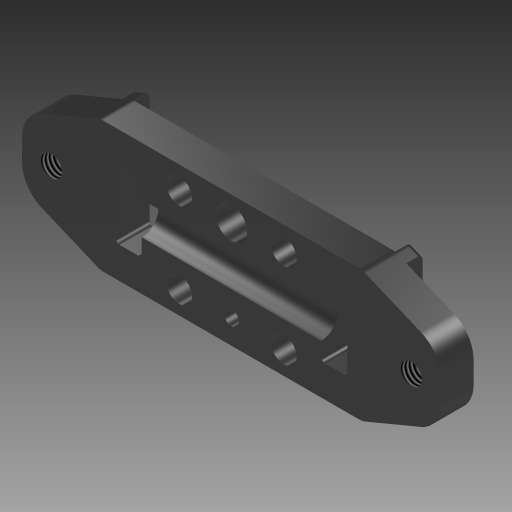
# Autodesk Inventor part: TTB Sliding Bearing Block Plate (SLIDE-001)
Saved by Autodesk Inventor 2023 (Build 270158000, 158)
## iProperties
Created: 2022-11-17
Part Number: TTB Sliding Bearing Block Plate (SLIDE-001)
Material: Aluminum 6061
Document SubType Name: Modeling
Designer: Max Boord
Mass: 26.5057 g
Surface Area: 60.4587 cm^2
Volume: 9.81693 cm^3
Density: 2.7 g/cm^3
Appearance: Glossy - Black
Author: Max Boord
Autodesk Inventor part; units mm, degrees
ref_plane "YZ Plane" through (0, 0, 0) normal (1, 0, 0) x (0, 1, 0)
ref_plane "XZ Plane" through (0, 0, 0) normal (0, 1, 0) x (-1, 0, 0)
ref_plane "XY Plane" through (0, 0, 0) normal (0, 0, 1) x (1, 0, 0)
sketch "Sketch1" plane through (0, 0, 0) normal (0, 0, 1) x (1, 0, 0)
  arc A0 (24.765, -12.7) -> (25.9862, -12.4558) centre (24.765, -9.525) ccw
  line L0 (25.9862, -12.4558) -> (36.7323, -7.9782)
  arc A1 (36.7323, -7.9782) -> (40.64, -2.1167) centre (34.29, -2.1167) ccw
  line L1 (40.64, -2.1167) -> (40.64, 2.1167)
  arc A2 (40.64, 2.1167) -> (36.7323, 7.9782) centre (34.29, 2.1167) ccw
  line L2 (36.7323, 7.9782) -> (25.9862, 12.4558)
  arc A3 (25.9862, 12.4558) -> (24.765, 12.7) centre (24.765, 9.525) ccw
  line L3 (24.765, 12.7) -> (-24.765, 12.7)
  arc A4 (-24.765, 12.7) -> (-25.9862, 12.4558) centre (-24.765, 9.525) ccw
  line L4 (-25.9862, 12.4558) -> (-36.7323, 7.9782)
  arc A5 (-36.7323, 7.9782) -> (-40.64, 2.1167) centre (-34.29, 2.1167) ccw
  line L5 (-40.64, 2.1167) -> (-40.64, -2.1167)
  arc A6 (-40.64, -2.1167) -> (-36.7323, -7.9782) centre (-34.29, -2.1167) ccw
  line L6 (-36.7323, -7.9782) -> (-25.9862, -12.4558)
  arc A7 (-25.9862, -12.4558) -> (-24.765, -12.7) centre (-24.765, -9.525) ccw
  line L7 (-24.765, -12.7) -> (24.765, -12.7)
  circle A8 centre (0, -7.9502) radius 1.4605
  circle A9 centre (-34.925, 0) radius 2.0193
  circle A10 centre (34.925, 0) radius 2.0193
  circle A11 centre (-10.16, 8.255) radius 2.4892
  circle A12 centre (-10.16, -8.255) radius 2.4892
  circle A13 centre (10.16, 8.255) radius 2.4892
  circle A14 centre (10.16, -8.255) radius 2.4892
  line L8 (17.399, -3.1979) -> (-17.399, -3.1979)
  line L9 (-17.399, -3.1979) -> (-17.399, -5.7785)
  arc A15 (-18.2245, -6.604) -> (-17.399, -5.7785) centre (-18.2245, -5.7785) ccw
  line L10 (-18.2245, -6.604) -> (-21.6535, -6.604)
  arc A16 (-22.479, -5.7785) -> (-21.6535, -6.604) centre (-21.6535, -5.7785) ccw
  line L11 (-22.479, -5.7785) -> (-22.479, 5.7785)
  arc A17 (-21.6535, 6.604) -> (-22.479, 5.7785) centre (-21.6535, 5.7785) ccw
  line L12 (-21.6535, 6.604) -> (-18.2245, 6.604)
  arc A18 (-17.399, 5.7785) -> (-18.2245, 6.604) centre (-18.2245, 5.7785) ccw
  line L13 (-17.399, 5.7785) -> (-17.399, 3.1979)
  line L14 (-17.399, 3.1979) -> (17.399, 3.1979)
  line L15 (17.399, 3.1979) -> (17.399, 5.7785)
  arc A19 (18.2245, 6.604) -> (17.399, 5.7785) centre (18.2245, 5.7785) ccw
  line L16 (18.2245, 6.604) -> (21.6535, 6.604)
  arc A20 (22.479, 5.7785) -> (21.6535, 6.604) centre (21.6535, 5.7785) ccw
  line L17 (22.479, 5.7785) -> (22.479, -5.7785)
  arc A21 (21.6535, -6.604) -> (22.479, -5.7785) centre (21.6535, -5.7785) ccw
  line L18 (21.6535, -6.604) -> (18.2245, -6.604)
  arc A22 (17.399, -5.7785) -> (18.2245, -6.604) centre (18.2245, -5.7785) ccw
  line L19 (17.399, -5.7785) -> (17.399, -3.1979)
  circle A23 centre (0, 7.9502) radius 3.048
  line L20 (-40.64, 0) -> (40.64, 0) construction
  line L21 (0, 7.9502) -> (0, -7.9502) construction
  line L22 (-10.16, 8.255) -> (10.16, -8.255) construction
  line L23 (-10.16, -8.255) -> (10.16, 8.255) construction
  line L24 (-34.925, 0) -> (0, 0) construction
  line L25 (0, 0) -> (34.925, 0) construction
  line L26 (-25.4, 12.6359) -> (-25.4, -12.6359)
  line L27 (-27.6098, -11.7792) -> (-27.6098, 11.7792)
  line L28 (27.6098, 11.7792) -> (27.6098, -11.7792)
  line L29 (25.4, -12.6359) -> (25.4, 12.6359)
  line L30 (-17.399, 3.1979) -> (-17.399, -3.1979)
  line L31 (17.399, 3.1979) -> (17.399, -3.1979)
  line L32 (0, 7.9502) -> (0, -7.9502) construction
  line L33 (-1.4605, 7.9502) -> (-1.4605, -7.9502)
  line L34 (1.4605, -7.9502) -> (1.4605, 7.9502)
  arc A24 (1.4605, 7.9502) -> (-1.4605, 7.9502) centre (0, 7.9502) ccw
  arc A25 (-1.4605, -7.9502) -> (1.4605, -7.9502) centre (0, -7.9502) ccw
  point P0 (0, 12.7)
  point P1 (0, -12.7)
  point P2 (0, -3.1979)
  point P3 (0, 3.1979)
  point P4 (-22.479, 0)
  point P5 (22.479, 0)
  dimension "d0" = 4.9784
  dimension "d1" = 69.85
  dimension "d2" = 25.4
  dimension "d3" = 81.28
  dimension "d4" = 16.51
  dimension "d5" = 20.32
  dimension "d6" = 15.9004
  dimension "d7" = 13.208
  dimension "d8" = 5.08
  dimension "d9" = 1.651
  dimension "d11" = 6.3958
  dimension "d12" = 44.958
  dimension "d13" = 4.0386
  dimension "d14" = 6.35
  dimension "d15" = 4.2333
  dimension "d16" = 49.53
  dimension "d17" = 3.175
  dimension "d18" = 2.921
  dimension "d19" = 6.096
  dimension "d21" = 50.8
  dimension "d22" = 2.2098
  constraints: 72 end point, 49 centre point, 40 point on circle, 36 tangent, 18 equal radius, 13 midpoint, 12 equal length, 7 horizontal, 6 point on line, 4 horizontal alignment, 4 parallel, 4 perpendicular, 4 vertical, 3 vertical alignment, 1 coincident, 1 collinear, 3 other
  measures "d0" diameter of A11
  measures "d1" distance of L25.end L24.start
  measures "d2" distance between parallel lines of L7 L3
  measures "d3" distance between parallel lines of L1 L5
  measures "d4" distance of L23.start L22.start
  measures "d5" distance of L23.end L22.start
  measures "d6" distance of L21.end L21.start
  measures "d7" distance between parallel lines of L10 L12
  measures "d8" distance between parallel lines of L13 L11
  measures "d9" diameter of A17
  measures "d11" distance between parallel lines of L14 L8
  measures "d12" distance between parallel lines of L11 L17
  measures "d13" diameter of A9
  measures "d14" radius of A2
  measures "d15" distance of L5.start L5.end
  measures "d16" distance of L3.start L3.end
  measures "d17" radius of A4
  measures "d18" diameter of A8
  measures "d19" diameter of A23
  measures "d21" distance between parallel lines of L29 L26
  measures "d22" distance between parallel lines of L29 L28
extrude "Extrusion1" add sketch "Sketch1" along normal blind 6.35 contours L7 A7 L26 A4 L3 A3 L29 A0 | L29 A3 L2 L28 L0 A0 | A7 L6 L27 L4 A4 L26 | L28 L2 A2 L1 A1 L0 | L6 A6 L5 A5 L4 L27 | A8 L33 L8 L34 | L34 L14 L31 L8 | L8 L33 L14 L34 | L8 L30 L14 L33 | L14 L33 A23 L34 | L34 A24 L33 A23 | A23 L33 A24 L34
extrude "Extrusion2" add sketch "Sketch1" against normal blind 3.175 contours L29 A3 L2 L28 L0 A0 | A7 L6 L27 L4 A4 L26
extrude "Extrusion3" cut sketch "Sketch1" against normal blind 3.1979 from surface at 6.35 contours L34 L14 L31 L8 | L8 L33 L14 L34 | L8 L30 L14 L33
full round fillet "Full Round Fillet1" first side at (-5.7997, -3.1979, 5.284) centre faces at (-5.7997, 1.066, 3.1521) second side at (5.7997, 3.1979, 5.284)
fillet "Fillet1" radius 1 8 edges at (25.6974, 12.56, -3.175) (26.798, 12.1175, -3.175) (25.6974, -12.56, -3.175) (26.798, -12.1175, -3.175) (-25.6974, 12.56, -3.175) (-26.798, 12.1175, -3.175) (-25.6974, -12.56, -3.175) (-26.798, -12.1175, -3.175)
extrude "Extrusion4" cut sketch "Sketch1" along normal blind 2.032 contours A8 | A8 L33 L8 L34 | L8 L33 L14 L34 | L14 L33 A23 L34 | A23 L33 A24 L34 picked at (0, 6.9342)
extrude "Extrusion6" cut sketch "Sketch1" against normal blind 4.318 from surface at 6.35 contours L34 A24 L33 A23 | A23 L33 A24 L34
thread "Thread1" size "10-32 UNF" class "2B" standard "ANSI Unified Screw Threads" full length
thread "Thread2" size "10-32 UNF" class "2B" standard "ANSI Unified Screw Threads" full length
equation "\"d27\" = 0.5 * d11"
body "Solid1"
